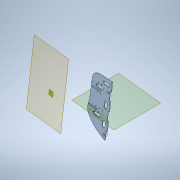
# Autodesk Inventor part: поперечная_поддержка
Saved by Autodesk Inventor 2020 (Build 240168000, 168)
## iProperties
Created: 2022-03-08
Part Number: поперечная_поддержка
Material: Типовые
Document SubType Name: Modeling
Designer: Администратор
Density: 1 g/cm^3
Appearance: Светло-синий стальной
Author: Администратор
Autodesk Inventor part; units mm, degrees
ref_plane "YZ Plane" through (0, 0, 0) normal (1, 0, 0) x (0, 1, 0)
ref_plane "XZ Plane" through (0, 0, 0) normal (0, 1, 0) x (-1, 0, 0)
ref_plane "XY Plane" through (0, 0, 0) normal (0, 0, 1) x (1, 0, 0)
ref_plane "РабПлоскость1" through (-276.9669, -64.4178, 0) normal (0, 0, 1) x (0.9934395, -0.1143588, 0)
sketch "Эскиз1" plane through (-276.9669, -64.4178, 0) normal (0, 0, 1) x (0.9934395, -0.1143588, 0)
  line L0 (291.0502, 248.6307) -> (221.0654, 248.6307) construction
  line L1 (221.0654, 248.6307) -> (209.9068, 234.7693) construction
  line L2 (209.9068, 234.7693) -> (196.6601, 234.7693) construction
  line L3 (196.6601, 234.7693) -> (196.6601, 175.7756) construction
  line L4 (196.6601, 175.7756) -> (196.6601, 136.8397) construction
  line L5 (196.6601, 136.8397) -> (196.6601, 100.2635) construction
  line L6 (196.6601, 100.2635) -> (185.4513, 58.9679) construction
  line L7 (185.4513, 58.9679) -> (192.5305, 32.4207) construction
  line L8 (192.5305, 32.4207) -> (238.9418, -16.2312) construction
  line L9 (238.9418, -16.2312) -> (291.0502, -35.7278) construction
  spline S0 degree 4 poles (291.0502, 248.6307) (221.0654, 248.6307) (209.9068, 234.7693) (196.6601, 234.7693) (196.6601, 175.7756) (196.6601, 136.8397) (196.6601, 100.2635) (185.4513, 58.9679) (192.5305, 32.4207) (238.9418, -16.2312) (291.0502, -35.7278) knots 1 1 1 1 1 2 3 4 5 6 7 8 8 8 8 8
  line L10 (291.0502, 248.6307) -> (291.0502, -35.7278)
  line L11 (295.0502, 248.6307) -> (291.0502, 248.6307) projected
  line L12 (291.0502, 248.6307) -> (591.0502, 248.6307) construction
  line L13 (291.0502, 248.6307) -> (-95.7817, 248.6307)
  line L14 (295.0502, -35.7278) -> (291.0502, -35.7278) projected
  line L15 (291.0502, -35.7278) -> (207.0762, -35.7278)
  line L16 (291.0502, -35.7278) -> (291.0502, -12.1198)
  line L17 (291.0508, -13.8678) -> (291.0488, -8.3678)
  line L18 (291.0507, -13.5698) -> (291.0496, -10.6698)
  line L19 (291.0507, -13.5698) -> (284.5507, -13.5698)
  line L20 (284.5507, -13.5698) -> (284.5507, -14.8698)
  line L21 (284.5507, -14.8698) -> (282.5507, -14.8698)
  line L22 (282.5507, -14.8698) -> (282.5507, -13.5698)
  line L23 (282.5507, -13.5698) -> (276.0507, -13.5698)
  line L24 (276.0507, -13.5698) -> (276.0507, -10.6698)
  line L25 (291.0507, -10.6698) -> (284.5507, -10.6698)
  line L26 (284.5507, -10.6698) -> (284.5507, -9.3698)
  line L27 (284.5507, -9.3698) -> (282.5507, -9.3698)
  line L28 (282.5507, -9.3698) -> (282.5507, -10.6698)
  line L29 (282.5507, -10.6698) -> (276.0507, -10.6698)
  line L30 (276.0507, -10.6698) -> (276.0507, -13.5698)
  line L31 (291.0502, 248.6307) -> (291.0502, 189.7587)
  line L32 (291.0502, 189.7587) -> (291.0502, -12.1198)
  line L33 (291.0507, 191.2087) -> (284.5507, 191.2087)
  line L34 (284.5507, 191.2087) -> (284.5507, 192.5087)
  line L35 (284.5507, 192.5087) -> (282.5507, 192.5087)
  line L36 (282.5507, 192.5087) -> (282.5507, 191.2087)
  line L37 (282.5507, 191.2087) -> (276.0507, 191.2087)
  line L38 (276.0507, 191.2087) -> (276.0507, 188.3087)
  line L39 (276.0507, 188.3087) -> (276.0507, 191.2087)
  line L40 (282.5507, 188.3087) -> (276.0507, 188.3087)
  line L41 (282.5507, 187.0087) -> (282.5507, 188.3087)
  line L42 (291.0507, 188.3087) -> (284.5507, 188.3087)
  line L43 (284.5507, 188.3087) -> (284.5507, 187.0087)
  line L44 (284.5507, 187.0087) -> (282.5507, 187.0087)
  point P0 (267.7832, 95.6688)
  point P1 (288.3259, -12.14)
  point P2 (291.0502, 191.2087)
  point P3 (291.0502, -13.5698)
  point P4 (276.0507, -10.6698)
  point P5 (291.0502, -10.6698)
  point P6 (291.0502, 188.3087)
  dimension "d116" = 23.608
  dimension "d135" = 2.9
  dimension "d136" = 6.5
  dimension "d137" = 1.3
  dimension "d138" = 2
  dimension "d139" = 58.872
  constraints: 66 end point, 6 horizontal, 5 point on line, 5 vertical, 3 perpendicular, 2 collinear, 1 coincident, 1 midpoint, 3 other
  measures "d116" distance of L9.end L16.end
  measures "d135" distance of L18.start L18.end
  measures "d136" distance of L18.start L19.end
  measures "d137" distance of L19.end L20.end
  measures "d138" distance of L20.end L21.end
  measures "d139" distance of L0.start L31.end
ref_plane "РабПлоскость3" through (10.9482, -108.3491, 1.5) normal (0.9934395, -0.1143588, 0) x (0, 0, -1)
sketch "Эскиз2" plane through (10.9482, -108.3491, 1.5) normal (0.9934395, -0.1143588, 0) x (0, 0, -1)
  line L0 (-0.5, 22.3828) -> (3.5, 22.3828)
  line L1 (3.5, 22.3828) -> (3.5, 69.7759)
  line L2 (3.5, 69.7759) -> (-0.5, 69.7759)
  line L3 (-0.5, 69.7759) -> (-0.5, 22.3828)
  line L4 (3.5, 164.562) -> (-0.5, 164.562)
  line L5 (-0.5, 164.562) -> (-0.5, 117.1689)
  line L6 (3.5, 117.1689) -> (3.5, 164.562)
  line L7 (-0.5, 117.1689) -> (3.5, 117.1689)
  line L8 (3.5, 259.3482) -> (-0.5, 259.3482)
  line L9 (-0.5, 259.3482) -> (-0.5, 211.9551)
  line L10 (3.5, 211.9551) -> (3.5, 259.3482)
  line L11 (-0.5, 211.9551) -> (3.5, 211.9551)
  line L12 (-0.5, -25.0103) -> (-0.5, 259.3482) projected
  line L13 (3.5, 259.3482) -> (3.5, -25.0103) projected
  line L14 (-0.5, -25.0103) -> (3.5, -25.0103) projected
  line L15 (3.5, 259.3482) -> (-0.5, 259.3482) projected
  line L16 (1.5, -25.0103) -> (1.5, 22.3828)
  line L17 (1.5, 69.7759) -> (1.5, 117.1689)
  point P0 (1.5, 106.3863)
  dimension "d110" = 94.7862
  constraints: 28 end point, 4 midpoint, 2 collinear, 2 equal length, 2 parallel, 2 point on line, 1 horizontal, 1 perpendicular, 1 vertical, 15 other
  measures "d110" distance of L2.end L4.end
extrude "Выдавливание2" add sketch "Эскиз2" along normal blind 6 contours L3 L2 L1 L0 | L5 L4 L6 L7 | L9 L8 L10 L11
sketch "Эскиз3" plane through (-276.9669, -64.4178, 0) normal (0, 0, 1) x (0.9934395, -0.1143588, 0)
  point P0 (267.7832, 95.6688)
sketch "Эскиз5" plane through (-276.9669, -64.4178, 0) normal (0, 0, 1) x (0.9934395, -0.1143588, 0)
  line L0 (291.0502, 173.347) -> (291.0502, 169.347) projected
  line L1 (246.0502, 173.347) -> (291.0502, 173.347) projected
  line L2 (246.0502, 173.347) -> (246.0502, 169.347) projected
  line L3 (291.0502, 169.347) -> (246.0502, 169.347) projected
  line L4 (246.0502, 173.347) -> (246.0502, 169.347)
  line L5 (186.6761, 173.347) -> (246.0502, 173.347)
  line L6 (186.6761, 173.347) -> (186.6761, 169.347)
  line L7 (186.6761, 169.347) -> (246.0502, 169.347)
  line L8 (246.0502, 173.347) -> (246.0502, 169.347)
  line L9 (186.6761, 173.347) -> (186.6761, 173.847)
  line L10 (186.6761, 173.847) -> (246.0502, 173.847)
  line L11 (246.0502, 173.847) -> (246.0502, 173.347)
  line L12 (246.0502, 169.347) -> (246.0502, 168.847)
  line L13 (246.0502, 168.847) -> (186.6761, 168.847)
  line L14 (186.6761, 168.847) -> (186.6761, 169.347)
  point P0 (267.7832, 95.6688)
  dimension "d14" = 0.5
  dimension "d15" = 0.5
  constraints: 22 end point, 4 perpendicular, 4 vertical, 2 collinear, 1 parallel
  measures "d14" distance of L5.start L9.end
  measures "d15" distance of L2.end L12.end
ref_plane "РабПлоскость7" through (-276.9669, -64.4178, -2) normal (0, 0, -1) x (-0.9934395, 0.1143588, 0)
sketch "Эскиз6" plane through (-276.9669, -64.4178, -2) normal (0, 0, -1) x (-0.9934395, 0.1143588, 0)
  line L0 (-291.0502, 201.2376) -> (-291.0502, 153.8445) projected
  line L1 (-291.0502, 248.6307) -> (-297.0502, 248.6307) projected
  line L2 (-297.0502, 201.2376) -> (-297.0502, 248.6307) projected
  line L3 (-291.0502, 201.2376) -> (-297.0502, 201.2376) projected
  line L4 (-291.0502, 153.8445) -> (-297.0502, 153.8445) projected
  line L5 (-297.0502, 106.4514) -> (-297.0502, 153.8445) projected
  line L6 (-291.0502, 106.4514) -> (-297.0502, 106.4514) projected
  line L7 (-291.0502, 106.4514) -> (-291.0502, 59.0584) projected
  line L8 (-291.0502, 59.0584) -> (-297.0502, 59.0584) projected
  line L9 (-297.0502, 11.6653) -> (-297.0502, 59.0584) projected
  line L10 (-291.0502, 11.6653) -> (-297.0502, 11.6653) projected
  line L11 (-291.0502, 11.6653) -> (-291.0502, -35.7278) projected
  point P0 (-267.7832, 95.6688)
  constraints: 1 vertical alignment
ref_plane "РабПлоскость2" through (1.8532, -16.6155, -86.2852) normal (-0.1143588, -0.9934395, 0) x (0, 0, 1)
sketch "Эскиз8" plane through (1.8532, -16.6155, -86.2852) normal (-0.1143588, -0.9934395, 0) x (0, 0, 1)
  line L0 (88.2852, 35.4303) -> (84.2852, 35.4303) projected
  line L1 (84.2852, 35.4303) -> (84.2852, 89.0995)
  line L2 (84.2852, 89.0995) -> (88.2852, 89.0995)
  line L3 (88.2852, 89.0995) -> (88.2852, 35.4303)
  point P0 (86.2852, 3.7412)
  constraints: 6 end point, 2 perpendicular, 1 vertical
extrude "Выдавливание8" cut sketch "Эскиз5" against normal through all both and the other way through all contours L2 L7 L6 L5
ref_plane "РабПлоскость8" through (-276.9669, -64.4178, -2) normal (0, 0, -1) x (-0.9934395, 0.1143588, 0)
sketch "Эскиз9" plane through (-276.9669, -64.4178, -2) normal (0, 0, -1) x (-0.9934395, 0.1143588, 0)
  line L0 (-291.0502, 201.2376) -> (-291.0502, -35.7278) projected
  line L1 (-291.0502, -35.7278) -> (-291.0502, 11.6653) projected
  line L2 (-291.0502, 248.6307) -> (-291.0502, 173.6307)
  line L3 (-250.374, 197.2593) -> (-229.374, 197.2593)
  line L4 (-222.374, 190.2593) -> (-222.374, 189.2593)
  line L5 (-229.374, 182.2593) -> (-250.374, 182.2593)
  line L6 (-257.374, 189.2593) -> (-257.374, 190.2593)
  arc A0 (-250.374, 197.2593) -> (-257.374, 190.2593) centre (-250.374, 190.2593) ccw
  arc A1 (-222.374, 190.2593) -> (-229.374, 197.2593) centre (-229.374, 190.2593) ccw
  arc A2 (-229.374, 182.2593) -> (-222.374, 189.2593) centre (-229.374, 189.2593) ccw
  arc A3 (-257.374, 189.2593) -> (-250.374, 182.2593) centre (-250.374, 189.2593) ccw
  line L7 (-246.0502, 173.347) -> (-196.6732, 173.347) projected
  line L8 (-236.094, 82.3742) -> (-191.8627, 82.3742) projected
  line L9 (-246.0502, 169.347) -> (-246.0502, 173.347) projected
  line L10 (-291.0502, -35.7278) -> (-291.0502, 11.6653) projected
  line L11 (-291.0502, 168.3876) -> (-291.0502, 108.6859)
  line L12 (-270.0097, 135.2593) -> (-270.0097, 114.2593)
  line L13 (-277.0097, 107.2593) -> (-278.0097, 107.2593)
  line L14 (-285.0097, 114.2593) -> (-285.0097, 135.2593)
  line L15 (-278.0097, 142.2593) -> (-277.0097, 142.2593)
  arc A4 (-285.0097, 114.2593) -> (-278.0097, 107.2593) centre (-278.0097, 114.2593) ccw
  arc A5 (-277.0097, 107.2593) -> (-270.0097, 114.2593) centre (-277.0097, 114.2593) ccw
  arc A6 (-278.0097, 142.2593) -> (-285.0097, 135.2593) centre (-278.0097, 135.2593) ccw
  arc A7 (-270.0097, 135.2593) -> (-277.0097, 142.2593) centre (-277.0097, 135.2593) ccw
  line L16 (-291.0502, 128.1496) -> (-171.8864, 128.1496) construction
  line L17 (-250.3741, 49.6336) -> (-229.3741, 49.6336)
  line L18 (-222.3741, 56.6336) -> (-222.3741, 57.6336)
  line L19 (-229.3741, 64.6336) -> (-250.3741, 64.6336)
  line L20 (-257.3741, 57.6336) -> (-257.3741, 56.6336)
  arc A8 (-257.3741, 56.6336) -> (-250.3741, 49.6336) centre (-250.3741, 56.6336) ccw
  arc A9 (-229.3741, 49.6336) -> (-222.3741, 56.6336) centre (-229.3741, 56.6336) ccw
  arc A10 (-222.3741, 57.6336) -> (-229.3741, 64.6336) centre (-229.3741, 57.6336) ccw
  arc A11 (-250.3741, 64.6336) -> (-257.3741, 57.6336) centre (-250.3741, 57.6336) ccw
  line L21 (-291.0502, 211.1307) -> (-160.6056, 211.1307) construction
  line L22 (-225.8279, 211.1307) -> (-225.8279, 168.3876) construction
  line L23 (-291.0502, 168.3876) -> (-297.0502, 168.3876) projected
  line L24 (-225.8279, 189.7591) -> (-291.0502, 189.7591) construction
  line L25 (-191.259, 78.3742) -> (-236.094, 78.3742)
  line L26 (-236.094, 78.3742) -> (-236.094, 82.3742)
  line L27 (-196.6645, 169.347) -> (-246.0502, 169.347)
  line L28 (-246.0502, 173.347) -> (-246.0502, 169.347)
  line L29 (-246.0502, 173.347) -> (-196.6732, 173.347)
  line L30 (-191.8627, 82.3742) -> (-191.259, 78.3742)
  line L31 (-281.5047, 230.6541) -> (-260.5047, 230.6541)
  line L32 (-253.5047, 223.6541) -> (-253.5047, 222.6541)
  line L33 (-260.5047, 215.6541) -> (-281.5047, 215.6541)
  line L34 (-288.5047, 222.6541) -> (-288.5047, 223.6541)
  arc A12 (-281.5047, 230.6541) -> (-288.5047, 223.6541) centre (-281.5047, 223.6541) ccw
  arc A13 (-253.5047, 223.6541) -> (-260.5047, 230.6541) centre (-260.5047, 223.6541) ccw
  arc A14 (-260.5047, 215.6541) -> (-253.5047, 222.6541) centre (-260.5047, 222.6541) ccw
  arc A15 (-288.5047, 222.6541) -> (-281.5047, 215.6541) centre (-281.5047, 222.6541) ccw
  line L35 (-78.1939, 79.3742) -> (-385.2661, 79.3742) projected
  line L36 (-270.0097, 23.4891) -> (-270.0097, 44.4891)
  line L37 (-277.0097, 51.4891) -> (-278.0097, 51.4891)
  line L38 (-285.0097, 44.4891) -> (-285.0097, 23.4891)
  line L39 (-278.0097, 16.4891) -> (-277.0097, 16.4891)
  arc A16 (-278.0097, 51.4891) -> (-285.0097, 44.4891) centre (-278.0097, 44.4891) ccw
  arc A17 (-270.0097, 44.4891) -> (-277.0097, 51.4891) centre (-277.0097, 44.4891) ccw
  arc A18 (-285.0097, 23.4891) -> (-278.0097, 16.4891) centre (-278.0097, 23.4891) ccw
  arc A19 (-277.0097, 16.4891) -> (-270.0097, 23.4891) centre (-277.0097, 23.4891) ccw
  point P0 (-267.7832, 95.6688)
  point P1 (-291.0502, 48.9842)
  point P2 (-257.374, 189.7593)
  point P3 (-224.8279, 190.7591)
  point P4 (-256.374, 190.7593)
  dimension "d28" = 75
  dimension "d29" = 7
  dimension "d41" = 65.035
  dimension "d46" = 35
  dimension "d67" = 1
  dimension "d130" = 7
  dimension "d131" = 35
  dimension "d132" = 1
  constraints: 64 end point, 40 point on circle, 20 centre point, 16 tangent, 12 symmetric about line, 7 horizontal, 6 equal radius, 5 perpendicular, 4 midpoint, 4 parallel, 4 point on line, 2 vertical, 1 collinear, 7 other
  measures "d28" distance of L2.start L2.end
  measures "d29" radius of A0
  measures "d41" distance of L3.start L12.start
  measures "d46" distance between parallel lines of L4 L6
  measures "d67" distance of L4.start L4.end
  measures "d130" radius of A12
  measures "d131" distance between parallel lines of L32 L34
  measures "d132" distance of L32.start L32.end
ref_plane "РабПлоскость6" through (-276.9669, -64.4178, -2) normal (0, 0, -1) x (-0.9934395, 0.1143588, 0)
sketch "Эскиз10" plane through (-276.9669, -64.4178, -2) normal (0, 0, -1) x (-0.9934395, 0.1143588, 0)
  line L0 (-230.0371, 169.347) -> (-246.0371, 169.347) construction
  line L1 (-238.0371, 191.7298) -> (-238.0371, 94.1825) construction
  line L2 (-196.6645, 169.347) -> (-246.0502, 169.347) projected
  line L3 (-228.5371, 163.347) -> (-230.5371, 163.347)
  line L4 (-230.5371, 163.347) -> (-230.5371, 159.347)
  line L5 (-230.5371, 159.347) -> (-228.5371, 159.347)
  line L6 (-228.5371, 159.347) -> (-228.5371, 163.347)
  line L7 (-247.5371, 163.347) -> (-245.5371, 163.347)
  line L8 (-245.5371, 163.347) -> (-245.5371, 159.347)
  line L9 (-245.5371, 159.347) -> (-247.5371, 159.347)
  line L10 (-247.5371, 159.347) -> (-247.5371, 163.347)
  line L11 (-196.6732, 173.347) -> (-246.0502, 173.347) projected
  line L12 (-247.5371, 93.347) -> (-245.5371, 93.347)
  line L13 (-245.5371, 93.347) -> (-245.5371, 89.347)
  line L14 (-245.5371, 89.347) -> (-247.5371, 89.347)
  line L15 (-247.5371, 89.347) -> (-247.5371, 93.347)
  line L16 (-230.5371, 93.347) -> (-230.5371, 89.347)
  line L17 (-228.5371, 93.347) -> (-230.5371, 93.347)
  line L18 (-230.5371, 89.347) -> (-228.5371, 89.347)
  line L19 (-228.5371, 89.347) -> (-228.5371, 93.347)
  line L20 (-236.094, 82.3742) -> (-191.8627, 82.3742) projected
  line L21 (-94.3517, 79.3742) -> (-382.4998, 79.3742) projected
  line L22 (-232.5371, 74.6336) -> (-230.5371, 74.6336)
  line L23 (-230.5371, 74.6336) -> (-230.5371, 70.6336)
  line L24 (-230.5371, 70.6336) -> (-232.5371, 70.6336)
  line L25 (-232.5371, 70.6336) -> (-232.5371, 74.6336)
  line L26 (-232.5371, 74.6336) -> (-230.5371, 70.6336) construction
  line L27 (-230.5371, 74.6336) -> (-232.5371, 70.6336) construction
  line L28 (-247.5371, 74.6336) -> (-245.5371, 74.6336)
  line L29 (-245.5371, 74.6336) -> (-245.5371, 70.6336)
  line L30 (-245.5371, 70.6336) -> (-247.5371, 70.6336)
  line L31 (-247.5371, 70.6336) -> (-247.5371, 74.6336)
  line L32 (-247.5371, 74.6336) -> (-245.5371, 70.6336) construction
  line L33 (-245.5371, 74.6336) -> (-247.5371, 70.6336) construction
  line L34 (-250.3741, 64.6336) -> (-229.3741, 64.6336) projected
  line L35 (-246.5371, 72.6336) -> (-231.5371, 72.6336) construction
  line L36 (-229.3741, 64.6336) -> (-250.3741, 64.6336) projected
  arc A0 (-222.3741, 57.6336) -> (-229.3741, 64.6336) centre (-229.3741, 57.6336) ccw projected
  arc A1 (-229.3741, 49.6336) -> (-222.3741, 56.6336) centre (-229.3741, 56.6336) ccw projected
  line L37 (-222.3741, 57.6336) -> (-222.3741, 56.6336) projected
  line L38 (-203.548, 59.6336) -> (-201.548, 59.6336)
  line L39 (-201.548, 59.6336) -> (-201.548, 55.6336)
  line L40 (-201.548, 55.6336) -> (-203.548, 55.6336)
  line L41 (-203.548, 55.6336) -> (-203.548, 59.6336)
  line L42 (-233.0371, 75.6336) -> (-231.0371, 71.6336) construction
  line L43 (-231.0371, 75.6336) -> (-233.0371, 71.6336) construction
  line L44 (-220.548, 59.6336) -> (-218.548, 59.6336)
  line L45 (-218.548, 59.6336) -> (-218.548, 55.6336)
  line L46 (-218.548, 55.6336) -> (-220.548, 55.6336)
  line L47 (-220.548, 55.6336) -> (-220.548, 59.6336)
  line L48 (-243.0371, 75.6336) -> (-241.0371, 71.6336) construction
  line L49 (-241.0371, 75.6336) -> (-243.0371, 71.6336) construction
  line L50 (-242.0371, 73.6336) -> (-232.0371, 73.6336) construction
  line L51 (-247.5371, 206.2593) -> (-245.5371, 206.2593)
  line L52 (-245.5371, 206.2593) -> (-245.5371, 202.2593)
  line L53 (-245.5371, 202.2593) -> (-247.5371, 202.2593)
  line L54 (-247.5371, 202.2593) -> (-247.5371, 206.2593)
  line L55 (-230.5371, 206.2593) -> (-228.5371, 206.2593)
  line L56 (-228.5371, 206.2593) -> (-228.5371, 202.2593)
  line L57 (-228.5371, 202.2593) -> (-230.5371, 202.2593)
  line L58 (-230.5371, 202.2593) -> (-230.5371, 206.2593)
  line L59 (-250.374, 197.2593) -> (-229.374, 197.2593) projected
  line L60 (-203.548, 192.6797) -> (-201.548, 192.6797)
  line L61 (-201.548, 188.6797) -> (-203.548, 188.6797)
  line L62 (-203.548, 188.6797) -> (-203.548, 192.6797)
  line L63 (-201.548, 192.6797) -> (-201.548, 188.6797)
  line L64 (-218.548, 192.6797) -> (-218.548, 188.6797)
  line L65 (-220.548, 192.6797) -> (-218.548, 192.6797)
  line L66 (-218.548, 188.6797) -> (-220.548, 188.6797)
  line L67 (-220.548, 188.6797) -> (-220.548, 192.6797)
  point P0 (-267.7832, 95.6688)
  point P1 (-238.0371, 169.347)
  point P2 (-238.0371, 121.7298)
  point P3 (-231.5371, 74.6336)
  point P4 (-247.5371, 72.6336)
  point P5 (-232.0371, 75.6336)
  point P6 (-243.0371, 73.6336)
  dimension "d47" = 2
  dimension "d48" = 4
  dimension "d49" = 15
  dimension "d53" = 70
  dimension "d64" = 6
  dimension "d66" = 9.9727
  dimension "d73" = 4
  dimension "d74" = 2
  dimension "d79" = 15
  dimension "d81" = 4
  dimension "d82" = 2
  dimension "d87" = 15
  dimension "d88" = 5
  dimension "d89" = 15
  dimension "d100" = 4
  dimension "d101" = 2
  dimension "d102" = 15
  constraints: 118 end point, 20 parallel, 11 midpoint, 10 equal length, 10 perpendicular, 9 horizontal, 5 collinear, 4 symmetric about line, 3 point on line, 1 vertical, 17 other
  measures "d47" distance of L3.start L3.end
  measures "d48" distance of L3.end L4.end
  measures "d49" distance between parallel lines of L8 L4
  measures "d53" distance of L8.end L13.end
  measures "d64" distance between parallel lines of L0 L7
  measures "d66" distance between parallel lines of L21 L14
  measures "d73" distance of L22.end L23.end
  measures "d74" distance of L22.start L22.end
  measures "d79" distance of L35.start L35.end
  measures "d81" distance of L38.end L40.start
  measures "d82" distance of L38.start L38.end
  measures "d87" distance between parallel lines of L41 L45
  measures "d88" distance between parallel lines of L59 L53
  measures "d89" distance between parallel lines of L58 L52
  measures "d100" distance of L60.end L61.start
  measures "d101" distance of L60.start L60.end
  measures "d102" distance between parallel lines of L62 L64
ref_plane "РабПлоскость5" through (-276.9669, -64.4178, -2) normal (0, 0, -1) x (-0.9934395, 0.1143588, 0)
sketch "Эскиз12" plane through (-276.9669, -64.4178, -2) normal (0, 0, -1) x (-0.9934395, 0.1143588, 0)
  point P0 (-267.7832, 95.6688)
extrude "Выдавливание16" cut sketch "Эскиз10" against normal blind 10 contours L38 L39 L40 L41 | L44 L45 L46 L47
sketch "Эскиз13" plane through (16.9088, -109.0353, 1.5) normal (0.9934395, -0.1143588, 0) x (0, 0, -1)
  line L0 (-0.5, 0) -> (3.5, 0) projected
  line L1 (-0.5005, 1.5) -> (3.5005, 1.5)
  line L2 (-0.5, 59.7017) -> (-0.5, 0) projected
  line L3 (3.5, 0) -> (3.5, 59.7017) projected
  point P0 (1.5, 106.3863)
  point P1 (3.5, 1.5)
  point P2 (-0.5, 1.5)
  constraints: 2 end point, 1 horizontal, 2 other
extrude "Выдавливание20" cut sketch "Эскиз13" against normal blind 6
ref_plane "РабПлоскость9" through (-276.9669, -64.4178, -2) normal (0, 0, -1) x (-0.9934395, 0.1143588, 0)
sketch "Эскиз14" plane through (-276.9669, -64.4178, -2) normal (0, 0, -1) x (-0.9934395, 0.1143588, 0)
  point P0 (-267.7832, 95.6688)
sketch "Эскиз15" plane through (41.1477, 101.5293, -2) normal (0, 0, -1) x (-0.9934395, 0.1143588, 0)
  line L0 (100.377, -27.8906) -> (51, -27.8906) projected
  line L1 (67.0131, -31.8906) -> (51.0131, -31.8906) construction
  line L2 (100.3857, -31.8906) -> (51, -31.8906) projected
  spline S0 degree 4 poles (6, -236.9654) (58.1084, -217.4688) (104.5196, -168.8169) (111.5989, -142.2697) (100.39, -100.9741) (100.39, -64.3979) (100.39, -25.462) (100.39, 33.5317) (87.1433, 33.5317) (75.9848, 47.3931) (6, 47.3931) knots 0 0 0 0 0 0.142857 0.285714 0.428571 0.571429 0.714286 0.857143 1 1 1 1 1 projected
  line L3 (60.9561, -118.8634) -> (105.1875, -118.8634) projected
  line L4 (51, -27.8906) -> (51, -31.8906)
  line L5 (60.9561, -118.8634) -> (60.9129, -121.8673)
  point P0 (29.267, -105.5688)
  constraints: 4 end point, 1 perpendicular, 1 other
extrude "Выдавливание25" cut sketch "Эскиз15" against normal blind 4
extrude "Выдавливание26" cut sketch "Эскиз9" against normal blind 4 contours L8 L30 L35 L26 | L35 L30 L25 L26
sketch "Эскиз16" plane through (41.1477, 101.5293, -2) normal (0, 0, -1) x (-0.9934395, 0.1143588, 0)
  point P0 (29.267, -105.5688)
extrude "Выдавливание28" add sketch "Эскиз1" along normal mid plane 4 contours L10 L33 L34 L35 L36 L37 L38 L40 L41 L44 L43 L42 L25 L26 L27 L28 L29 L24 L23 L22 L21 L20 L19 S0
extrude "Выдавливание29" cut sketch "Эскиз10" against normal blind 4
extrude "Выдавливание30" cut sketch "Эскиз9" against normal blind 4 contours L3 A1 L4 A2 L5 A3 L6 A0 | L8 L30 L35 L26 | L35 L30 L25 L26 | L12 A5 L13 A4 L14 A6 L15 A7 | A8 L20 A11 L19 A10 L18 A9 L17 | L31 A13 L32 A14 L33 A15 L34 A12
extrude "Выдавливание31" cut sketch "Эскиз15" against normal blind 4
extrude "Выдавливание33" cut sketch "Эскиз9" against normal blind 4 contours A19 L39 A18 L38 A16 L37 A17 L36
